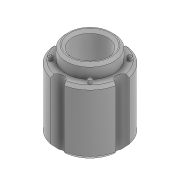
# Autodesk Inventor part: centrifugetool_5mm_tubecap_v2
Saved by Autodesk Inventor 2021.2 (Build 252289000, 289)
## iProperties
Created: 2021-12-08
Part Number: centrifugetool_5mm_tubecap_v2
Material: Generic
Document SubType Name: Modeling
Designer: tomos
Density: 1 g/cm^3
Appearance: Smooth - Medium Gray
Author: tomos
Autodesk Inventor part; units mm, degrees
ref_plane "YZ Plane" through (0, 0, 0) normal (1, 0, 0) x (0, 1, 0)
ref_plane "XZ Plane" through (0, 0, 0) normal (0, 1, 0) x (-1, 0, 0)
ref_plane "XY Plane" through (0, 0, 0) normal (0, 0, 1) x (1, 0, 0)
sketch "Sketch1" plane through (0, 0, 0) normal (0, 0, 1) x (1, 0, 0)
  line L0 (0, 0) -> (42.0469, 0) construction
  line L1 (0, 0) -> (0, 27.7015) construction
  arc A0 (0, -6.6) -> (6.5875, 0.406) centre (0, 0) ccw
  line L2 (6.5875, 0.406) -> (6.5875, 16)
  line L3 (6.5875, 16) -> (9, 16)
  line L4 (9, 16) -> (9, 21)
  line L5 (9, 21) -> (12.5, 21)
  line L6 (12.5, 21) -> (12.5, -8.6)
  line L7 (12.5, -8.6) -> (0, -8.6)
  line L8 (0, -8.6) -> (0, -6.6)
  line L9 (9, 16) -> (6.5875, 16)
  line L10 (6.5875, 16) -> (6.5875, 21)
  line L11 (6.5875, 21) -> (9, 21)
  line L12 (9, 21) -> (9, 16)
  line L13 (12.5, 16) -> (9, 16)
  line L14 (2, -8.6) -> (0, -8.6)
  line L15 (0, -8.6) -> (0, -6.6)
  dimension "d0" = 13.2
  dimension "d2" = 5
  dimension "d3" = 9
  dimension "d4" = 12.5
  dimension "d5" = 6.5875
  dimension "d6" = 2
  dimension "d35" = 16
  constraints: 32 end point, 6 perpendicular, 4 collinear, 3 horizontal, 2 parallel, 2 point on circle, 2 point on line, 2 vertical, 1 centre point, 1 coincident
  measures "d0" diameter of A0
  measures "d2" distance between parallel lines of L3 L5
  measures "d3" distance between parallel lines of L1 L4
  measures "d4" distance between parallel lines of L1 L6
  measures "d5" distance between parallel lines of L2 L1
  measures "d6" distance from line of L8.end L7
  measures "d35" distance between parallel lines of L0 L13
revolve "Revolution1" add sketch "Sketch1" angle 360 about axis through (0, 0, 0) along (0, 1, 0) contours A0 L2 L3 L13 L6 L7 L8 | L10 L11 L4 L3
chamfer "Chamfer1" distance 2 angle 45 1 edges at (-12.5, -8.6, 0)
chamfer "Chamfer3" distance 1 angle 45 3 edges at (-9, 21, 0) (-12.5, 16, 0) (-6.5875, 21, 0)
sketch "Sketch2" plane through (0, 16, 0) normal (0, 1, 0) x (1, 0, 0)
  circle A0 centre (0, 0) radius 10.5 construction
  line L0 (0, 0) -> (0, 17.3905) construction
  line L1 (0, 0) -> (14.2747, 14.2747) construction
  circle A1 centre (7.4246, 7.4246) radius 0.75
  circle A2 centre (0, 0) radius 12.5 projected
  circle A3 centre (0, 0) radius 12.5
  circle A4 centre (0, 12.5) radius 2.5
  point P0 (-2.4875, 12.25)
  point P1 (2.4875, 12.25)
  dimension "d17" = 21
  dimension "d29" = 25
  dimension "d18" = 45
  dimension "d19" = 1.5
  dimension "d28" = 5
  constraints: 4 end point, 2 centre point, 2 coincident, 2 point on line, 1 vertical, 1 vertical alignment, 5 other
  measures "d18" angle of L1 L0
  measures "d19" diameter of A1
  measures "d28" diameter of A4
extrude "Extrusion1" add sketch "Sketch2" along normal blind 1.5 contours A1
chamfer "Chamfer4" distance 0.35 angle 45 1 edges at (6.6746, 17.5, -7.4246)
extrude "Extrusion2" cut sketch "Sketch2" against normal through all contours A4 A2 picked at (0, 11.6481)
pattern_circular "Circular Pattern2" count 4 over 360 about axis through (0, -10, 0) along (0, 1, 0) of "Extrusion1", "Extrusion2", "Chamfer4"
sketch "Sketch3" plane through (0, -8.6, -12.5) normal (0, -1, 0) x (1, 0, 0)
  circle A0 centre (0, 12.5) radius 1.5
  dimension "d37" = 3
  constraints: 1 centre point, 1 coincident
  measures "d37" diameter of A0
extrude "Extrusion3" cut sketch "Sketch3" against normal through all
chamfer "Chamfer5" distance 1 angle 45 1 edges at (-1.5, -8.6, 0)
body "Solid1"
